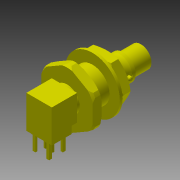
# Autodesk Inventor part: CJT-T-P-HH-RA-BH1
Saved by Autodesk Inventor 2014 SP2 (Build 180246200, 246)
## iProperties
Created: 2018-08-02
Part Number: CJT-T-P-HH-RA-BH1
Material: Generic
Catalog Web Link: www.cadenas.de
Description: CJT-BH Series-Circular RF Twinax Jack, Bulkhead Through-hole
Vendor: SAMTEC
Document SubType Name: Modeling
Designer: psadmin
Manufacturer: SAMTEC
Mass: 0.58128 g
Surface Area: 7.85862 cm^2
Volume: 0.58128 cm^3
Density: 1 g/cm^3
Appearance: PSOLRGB-255-255-0
Category: PARTsolutions
Company: SAMTEC
Title: CJT-T-P-HH-RA-BH1
Author: Cadenas PARTsolutions
Comments: Circular RF Twinax Jack, Bulkhead Through-hole
PSOL_IDENT_0: {$CADENAS_DATA\23d-libs\samtec\modelling\cjt\cjt-bh.prj},186 {VTYP=3D},{NB=CJT-T-P-HH-RA-BH1},{LINA=
PSOL_IDENT_1: CJT-T-P-HH-RA-BH1},{NN=CJT-BH Series},{DATE=26.10.2016 12:02:24},{GEOMDATE=19.09.2016 12:09:01},{VER
PSOL_IDENT_2: SION=},{LINEID=10},{WBVAR=PLOPT},{WBNUMERIC=}  {NB=CJT-T-P-HH-RA-BH1},{LINA=CJT-T-P-HH-RA-BH1},{KT=D
PSOL_IDENT_3: UMMY},{PN=CJT-T-P-HH-RA-BH1},{SERIES=CJT-BH},{GEN=-T: Terminal},{TYPE=-P: PCB},{PLOPT=HH},{PLOPTALG=
PSOL_IDENT_4: 'HH','-HH: Heavy Gold / Heavy Gold 30 µ\" Au / 50 µ\" Ni Min on Pin 30 µ\" Au / 50 µ\" Ni Min on Ou
PSOL_IDENT_5: ter Contact','GF','Non-standard option - Please contact SAMTEC: -GF: Gold / Flash Gold 10 µ\" Au / 5
PSOL_IDENT_6: 0 µ\" Ni Min on Pin 3 µ\" Au / 50 µ\" Ni Min on Outer Contact' },{ORI=-RA: Right Angle},{TERM=-BH1:
PSOL_IDENT_7: Bulkhead Through Hole}
NN: CJT-BH Series
NT: Circular RF Twinax Jack, Bulkhead Through-hole
NB: CJT-T-P-HH-RA-BH1
NBSYN: $PN.
LINA: CJT-T-P-HH-RA-BH1
PN: CJT-T-P-HH-RA-BH1
SERIES: CJT-BH
GEN: -T: Terminal
TYPE: -P: PCB
PLOPT: -HH: Heavy Gold / Heavy Gold 30 µ" Au / 50 µ" Ni Min on Pin 30 µ" Au / 50 µ" Ni Min on Outer Contact
ORI: -RA: Right Angle
TERM: -BH1: Bulkhead Through Hole
SUPPLIER: SAMTEC
ARTICLENO: CJT-T-P-HH-RA-BH1
BOMINFO: CJT-T-P-HH-RA-BH1
CREATOR: CADENAS GmbH
Autodesk Inventor part; units mm, degrees
ref_plane "YZ Plane" through (0, 0, 0) normal (1, 0, 0) x (0, 1, 0)
ref_plane "XZ Plane" through (0, 0, 0) normal (0, 1, 0) x (-1, 0, 0)
ref_plane "XY Plane" through (0, 0, 0) normal (0, 0, 1) x (1, 0, 0)
sketch "Sketch0" plane through (2.35, 0, 0) normal (1, 0, 0) x (0, 0, -1)
  line L0 (-2.417, -3.8772) -> (6.633, -3.8772)
  line L1 (6.633, -3.8772) -> (6.633, -0.1772)
  line L2 (6.633, -0.1772) -> (2.351, -0.1772)
  line L3 (2.351, -0.1772) -> (2.351, 0.8128)
  line L4 (2.351, 0.8128) -> (-2.417, 0.8128)
  line L5 (-2.417, 0.8128) -> (-2.417, -3.8772)
  constraints: 12 end point
extrude "Extrusion1" add sketch "Sketch0" against normal blind 4.7
sketch "Sketch2" plane through (0, 0, 0) normal (0, 0, 1) x (1, 0, 0)
  line L0 (-0.9949, 15.5369) -> (-0.4483, 14.5902)
  arc A0 (-0.38, 14.3352) -> (-0.4483, 14.5902) centre (-0.89, 14.3352) ccw
  line L1 (-0.38, 14.3352) -> (-0.38, 12.2628)
  arc A1 (-0.38, 12.2628) -> (0.38, 12.2628) centre (0, 12.2628) ccw
  line L2 (0.38, 12.2628) -> (0.38, 14.3352)
  arc A2 (0.4483, 14.5902) -> (0.38, 14.3352) centre (0.89, 14.3352) ccw
  line L3 (0.4483, 14.5902) -> (0.9949, 15.5369)
  line L4 (0.9949, 15.5369) -> (-0.9949, 15.5369)
  constraints: 10 end point, 6 point on circle, 3 centre point
sketch "Sketch1" plane through (0, 0, 0) normal (1, 0, 0) x (0, 0, -1)
  line L0 (0, 11.6728) -> (0, 0.8128)
  line L1 (0, 0.8128) -> (-2.35, 0.8128)
  line L2 (-2.35, 0.8128) -> (-2.35, 1.3128)
  line L3 (-2.35, 1.3128) -> (-5.05, 1.3128)
  line L4 (-5.05, 1.3128) -> (-5.3, 1.7458)
  line L5 (-5.3, 1.7458) -> (-5.3, 2.7128)
  line L6 (-5.3, 2.7128) -> (-4.867, 2.9628)
  line L7 (-4.867, 2.9628) -> (-4.025, 2.9628)
  line L8 (-4.025, 2.9628) -> (-4.025, 2.5678)
  line L9 (-4.025, 2.5678) -> (-3.175, 2.5678)
  line L10 (-3.175, 2.5678) -> (-3.175, 6.8128)
  line L11 (-3.175, 6.8128) -> (-4, 6.8128)
  line L12 (-4, 6.8128) -> (-4.6188, 7.1701)
  line L13 (-4.6188, 7.1701) -> (-4.6188, 8.4555)
  line L14 (-4.6188, 8.4555) -> (-4, 8.8128)
  line L15 (-4, 8.8128) -> (-2.35, 8.8128)
  line L16 (-2.35, 8.8128) -> (-2.35, 9.8878)
  arc A0 (-2.35, 9.8878) -> (-2.35, 11.0378) centre (-4.6766, 10.4628) ccw
  line L17 (-2.35, 11.0378) -> (-2.35, 11.6828)
  line L18 (-2.35, 11.6828) -> (-1.97, 11.6828)
  line L19 (-1.97, 11.6828) -> (-1.97, 14.9828)
  line L20 (-1.97, 14.9828) -> (-1.65, 14.9828)
  line L21 (-1.65, 14.9828) -> (-1.575, 14.5575)
  line L22 (-1.575, 14.5575) -> (-1.575, 11.6728)
  line L23 (-1.575, 11.6728) -> (0, 11.6728)
  line L24 (0, 11.6728) -> (0, 0.8128)
  constraints: 50 end point, 2 point on circle, 1 centre point
revolve "Revolution1" add sketch "Sketch1" angle 360 about axis through (0, 11.6728, 0) along (0, 1, 0)
sketch "Sketch3" plane through (0, 0, 0) normal (0, 0, 1) x (1, 0, 0)
  line L0 (0.635, 14.2828) -> (0.635, 11.6728)
  line L1 (0.635, 11.6728) -> (0.445, 11.6728)
  line L2 (0.445, 11.6728) -> (0.445, 14.0928)
  arc A0 (0.635, 14.2828) -> (0.445, 14.0928) centre (0.635, 14.0928) ccw
  line L3 (0.635, 14.2828) -> (0.635, 11.6728)
  constraints: 8 end point, 2 point on circle, 1 centre point
extrude "Extrusion2" cut sketch "Sketch2" against normal blind 1.97
sketch "Sketch4" plane through (0, 0, 0) normal (0, 0, 1) x (1, 0, 0)
  line L0 (-0.635, 14.2828) -> (-0.635, 11.6728)
  line L1 (-0.635, 11.6728) -> (-0.825, 11.6728)
  line L2 (-0.825, 11.6728) -> (-0.825, 14.0928)
  arc A0 (-0.635, 14.2828) -> (-0.825, 14.0928) centre (-0.635, 14.0928) ccw
  line L3 (-0.635, 14.2828) -> (-0.635, 11.6728)
  constraints: 8 end point, 2 point on circle, 1 centre point
revolve "Revolution2" add sketch "Sketch3" angle 360 about axis through (0.635, 14.2828, 0) along (0, 1, 0)
sketch "Sketch5" plane through (-2.2, 0, 0) normal (-1, 0, 0) x (0, 0, 1)
  circle A0 centre (0, 10.4628) radius 0.75
  constraints: 1 centre point
revolve "Revolution3" add sketch "Sketch4" angle 360 about axis through (-0.635, 14.2828, 0) along (0, 1, 0)
sketch "Sketch6" plane through (2.2, 0, 0) normal (1, 0, 0) x (0, 0, -1)
  circle A0 centre (0, 10.4628) radius 0.75
  constraints: 1 centre point
extrude "Extrusion3" cut sketch "Sketch5" along normal blind 0.15
sketch "Sketch7" plane through (0, 0, 0) normal (0, 0, 1) x (1, 0, 0)
  line L0 (2.79, 10.4628) -> (-2.79, 10.4628)
  line L1 (-2.79, 10.4628) -> (-2.79, 10.7128)
  line L2 (-2.79, 10.7128) -> (-2.69, 10.8128)
  line L3 (-2.69, 10.8128) -> (2.69, 10.8128)
  line L4 (2.69, 10.8128) -> (2.79, 10.7128)
  line L5 (2.79, 10.7128) -> (2.79, 10.4628)
  line L6 (2.79, 10.4628) -> (-2.79, 10.4628)
  constraints: 14 end point
extrude "Extrusion4" cut sketch "Sketch6" along normal blind 0.15
sketch "Sketch8" plane through (0, 2.9628, 0) normal (0, 1, 0) x (1, 0, 0)
  line L0 (-11.7464, 7.6127) -> (-11.7464, -9.9888)
  line L1 (-11.7464, -9.9888) -> (9.5951, -9.9888)
  line L2 (9.5951, -9.9888) -> (9.5951, 7.6127)
  line L3 (9.5951, 7.6127) -> (-11.7464, 7.6127)
  line L4 (-4.765, -2.7511) -> (0, -5.5021)
  line L5 (0, -5.5021) -> (4.765, -2.7511)
  line L6 (4.765, -2.7511) -> (4.765, 2.7511)
  line L7 (4.765, 2.7511) -> (0, 5.5021)
  line L8 (0, 5.5021) -> (-4.765, 2.7511)
  line L9 (-4.765, 2.7511) -> (-4.765, -2.7511)
  constraints: 20 end point
revolve "Revolution4" add sketch "Sketch7" angle 360 about axis through (2.79, 10.4628, 0) along (1, 0, 0)
sketch "Sketch9" plane through (0, 8.8128, 0) normal (0, 1, 0) x (1, 0, 0)
  line L0 (-10.8315, -11.6386) -> (13.3801, -11.6386)
  line L1 (13.3801, -11.6386) -> (13.3801, 10.789)
  line L2 (13.3801, 10.789) -> (-10.8315, 10.789)
  line L3 (-10.8315, 10.789) -> (-10.8315, -11.6386)
  line L4 (-4.6188, 0) -> (-2.3094, -4)
  line L5 (-2.3094, -4) -> (2.3094, -4)
  line L6 (2.3094, -4) -> (4.6188, 0)
  line L7 (4.6188, 0) -> (2.3094, 4)
  line L8 (2.3094, 4) -> (-2.3094, 4)
  line L9 (-2.3094, 4) -> (-4.6188, 0)
  constraints: 20 end point
extrude "Extrusion5" cut sketch "Sketch8" against normal blind 1.65
sketch "Sketch10" plane through (0, 0, -3.683) normal (0, 0, -1) x (-1, 0, 0)
  line L0 (-2.6213, -4.3652) -> (3.4207, -4.3652)
  line L1 (3.4207, -4.3652) -> (3.4207, 0.3295)
  line L2 (3.4207, 0.3295) -> (-2.6213, 0.3295)
  line L3 (-2.6213, 0.3295) -> (-2.6213, -4.3652)
  line L4 (0.89, -0.3772) -> (0.89, -0.7888)
  arc A0 (1.2384, -1.1372) -> (0.89, -0.7888) centre (0, -2.0272) ccw
  line L5 (1.2384, -1.1372) -> (1.65, -1.1372)
  line L6 (1.65, -1.1372) -> (1.65, -0.3772)
  line L7 (1.65, -0.3772) -> (0.89, -0.3772)
  line L8 (0.89, -3.6772) -> (1.65, -3.6772)
  line L9 (1.65, -3.6772) -> (1.65, -2.9172)
  line L10 (1.65, -2.9172) -> (1.2384, -2.9172)
  arc A1 (0.89, -3.2656) -> (1.2384, -2.9172) centre (0, -2.0272) ccw
  line L11 (0.89, -3.2656) -> (0.89, -3.6772)
  line L12 (-1.65, -0.3772) -> (-1.65, -1.1372)
  line L13 (-1.65, -1.1372) -> (-1.2384, -1.1372)
  arc A2 (-0.89, -0.7888) -> (-1.2384, -1.1372) centre (0, -2.0272) ccw
  line L14 (-0.89, -0.7888) -> (-0.89, -0.3772)
  line L15 (-0.89, -0.3772) -> (-1.65, -0.3772)
  line L16 (-1.65, -2.9172) -> (-1.65, -3.6772)
  line L17 (-1.65, -3.6772) -> (-0.89, -3.6772)
  line L18 (-0.89, -3.6772) -> (-0.89, -3.2656)
  arc A3 (-1.2384, -2.9172) -> (-0.89, -3.2656) centre (0, -2.0272) ccw
  line L19 (-1.2384, -2.9172) -> (-1.65, -2.9172)
  constraints: 40 end point, 8 point on circle, 4 centre point
extrude "Extrusion6" cut sketch "Sketch9" against normal blind 2
extrude "Extrusion7" cut sketch "Sketch10" along normal blind 0.25
sketch "Sketch11" plane through (0, 0, -3.683) normal (0, 0, -1) x (-1, 0, 0)
  circle A0 centre (-0.635, -2.0272) radius 0.255
  constraints: 1 centre point
sketch "Sketch12" plane through (0, 0, -3.933) normal (0, 0, -1) x (-1, 0, 0)
  line L0 (-2.434, -4.3856) -> (2.7387, -4.3856)
  line L1 (2.7387, -4.3856) -> (2.7387, -0.0557)
  line L2 (2.7387, -0.0557) -> (-2.434, -0.0557)
  line L3 (-2.434, -0.0557) -> (-2.434, -4.3856)
  line L4 (1.015, -0.5022) -> (1.015, -0.889)
  arc A0 (1.1382, -1.0122) -> (1.015, -0.889) centre (0, -2.0272) ccw
  line L5 (1.1382, -1.0122) -> (1.525, -1.0122)
  line L6 (1.525, -1.0122) -> (1.525, -0.5022)
  line L7 (1.525, -0.5022) -> (1.015, -0.5022)
  line L8 (1.015, -3.5522) -> (1.525, -3.5522)
  line L9 (1.525, -3.5522) -> (1.525, -3.0422)
  line L10 (1.525, -3.0422) -> (1.1382, -3.0422)
  arc A1 (1.015, -3.1654) -> (1.1382, -3.0422) centre (0, -2.0272) ccw
  line L11 (1.015, -3.1654) -> (1.015, -3.5522)
  line L12 (-1.525, -0.5022) -> (-1.525, -1.0122)
  line L13 (-1.525, -1.0122) -> (-1.1382, -1.0122)
  arc A2 (-1.015, -0.889) -> (-1.1382, -1.0122) centre (0, -2.0272) ccw
  line L14 (-1.015, -0.889) -> (-1.015, -0.5022)
  line L15 (-1.015, -0.5022) -> (-1.525, -0.5022)
  line L16 (-1.525, -3.0422) -> (-1.525, -3.5522)
  line L17 (-1.525, -3.5522) -> (-1.015, -3.5522)
  line L18 (-1.015, -3.5522) -> (-1.015, -3.1654)
  arc A3 (-1.1382, -3.0422) -> (-1.015, -3.1654) centre (0, -2.0272) ccw
  line L19 (-1.1382, -3.0422) -> (-1.525, -3.0422)
  constraints: 40 end point, 8 point on circle, 4 centre point
sketch "Sketch13" plane through (0, 0, 0) normal (0, 0, -1) x (-1, 0, 0)
  line L0 (0, 6.5128) -> (0, 6.0128)
  line L1 (0, 6.0128) -> (-5.075, 6.0128)
  line L2 (-5.075, 6.0128) -> (-5.075, 6.5128)
  line L3 (-5.075, 6.5128) -> (0, 6.5128)
  line L4 (0, 6.5128) -> (0, 6.0128)
  constraints: 10 end point
extrude "Extrusion8" cut sketch "Sketch12" along normal blind 2.7
extrude "Extrusion9" add sketch "Sketch11" along normal blind 2.7358
sketch "Sketch_1" plane through (0, 0, -3.683) normal (0, 0, -1) x (-1, 0, 0)
  circle A0 centre (0.635, -2.0272) radius 0.255
  constraints: 1 centre point
extrude "Extrusion10" add sketch "Sketch_1" along normal blind 2.7358
revolve "Revolution5" add sketch "Sketch13" angle 360 about axis through (0, 6.5128, 0) along (0, 1, 0)
body "Solid1"
